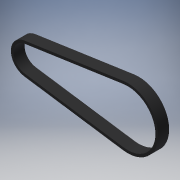
# Autodesk Inventor part: HTD5M 93 Belt
Saved by Autodesk Inventor 2019.4 (Build 234330000, 330)
## iProperties
Created: 2019-12-31
Part Number: HTD5M 93 Belt
Material: Rubber
Document SubType Name: Modeling
Designer: Mark
Density: 0.93 g/cm^3
Appearance: Rubber - Black
Mass: 23.2608 g
Surface Area: 172.302 cm^2
Volume: 25.0116 cm^3
Author: Mark
Autodesk Inventor part; units mm, degrees
ref_plane "YZ Plane" through (0, 0, 0) normal (1, 0, 0) x (0, 1, 0)
ref_plane "XZ Plane" through (0, 0, 0) normal (0, 1, 0) x (-1, 0, 0)
ref_plane "XY Plane" through (0, 0, 0) normal (0, 0, 1) x (1, 0, 0)
sketch "Sketch1" plane through (0, 0, 0) normal (0, 0, 1) x (1, 0, 0)
  arc A0 (-2.8807, 19.6399) -> (-2.8807, -19.6399) centre (0, 0) ccw
  arc A1 (131.6255, -39.3688) -> (131.6255, 39.3688) centre (137.4, 0) ccw
  line L0 (0, 0) -> (137.4, 0)
  line L1 (0, 0) -> (137.4, 0) construction
  line L2 (-2.8807, 19.6399) -> (131.6255, 39.3688)
  line L3 (-2.8807, -19.6399) -> (131.6255, -39.3688)
  arc A2 (131.9303, -37.291) -> (131.9303, 37.291) centre (137.4, 0) ccw
  line L4 (131.9303, 37.291) -> (-2.5759, 17.5621)
  arc A3 (-2.5759, 17.5621) -> (-2.5759, -17.5621) centre (0, 0) ccw
  line L5 (-2.5759, -17.5621) -> (131.9303, -37.291)
  arc A4 (131.4078, -40.8529) -> (131.4078, 40.8529) centre (137.4, 0) ccw
  line L6 (131.4078, 40.8529) -> (-3.0984, 21.124)
  arc A5 (-3.0984, 21.124) -> (-3.0984, -21.124) centre (0, 0) ccw
  line L7 (-3.0984, -21.124) -> (131.4078, -40.8529)
  dimension "d0" = 39.7
  dimension "d1" = 79.58
  dimension "d2" = 137.4
  dimension "d3" = 0
  dimension "d4" = 2.1
  dimension "d5" = 1.5
  constraints: 16 end point, 12 point on circle, 6 centre point, 4 tangent, 2 coincident, 2 horizontal, 1 collinear, 6 other
  measures "d0" diameter of A0
  measures "d1" diameter of A1
  measures "d2" distance of L0.start L0.end
  measures "d3" distance between parallel lines of L0 L1
  measures "d4" distance between parallel lines of L3 L5
  measures "d5" distance between parallel lines of L3 L7
extrude "Extrusion1" add sketch "Sketch1" along normal blind 15 contours L2 A1 L3 A0 | L7 A5 L6 A4
body "Solid1"
